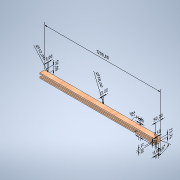
# Autodesk Inventor part: u_lange_Stange
Saved by Autodesk Inventor 2020.3 (Build 243373000, 373)
## iProperties
Created: 2020-09-30
Part Number: u_lange_Stange
Material: Birch
Document SubType Name: Modeling
Designer: Mara
Density: 0.512 g/cm^3
Appearance: Birch - Natural Medium Gloss
Author: Mara
Autodesk Inventor part; units mm, degrees
ref_plane "YZ Plane" through (0, 0, 0) normal (1, 0, 0) x (0, 1, 0)
ref_plane "XZ Plane" through (0, 0, 0) normal (0, 1, 0) x (-1, 0, 0)
ref_plane "XY Plane" through (0, 0, 0) normal (0, 0, 1) x (1, 0, 0)
sketch "Sketch1" plane through (0, 0, 0) normal (0, 0, 1) x (1, 0, 0)
  line L0 (-600, -25) -> (600, -25)
  line L1 (600, -25) -> (600, 25)
  line L2 (600, 25) -> (-600, 25)
  line L3 (-600, 25) -> (-600, -25)
  line L4 (-600, -25) -> (600, 25) construction
  line L5 (600, -25) -> (-600, 25) construction
  point P0 (0, 0)
  dimension "d0" = 1200
  dimension "d1" = 50
  constraints: 12 end point, 2 midpoint, 2 parallel, 1 horizontal, 1 perpendicular
  measures "d0" distance of L2.end L1.end
  measures "d1" distance of L1.end L0.end
extrude "Extrusion1" add sketch "Sketch1" along normal blind 50
sketch "Sketch2" plane through (0, 0, 0) normal (0, 0, -1) x (-1, 0, 0)
  circle A0 centre (0, 0) radius 9
  circle A1 centre (570, 0) radius 6
  line L0 (600, 25) -> (600, -25) projected
  line L1 (-600, 25) -> (600, 25) projected
  dimension "d13" = 18
  dimension "d20" = 30
  dimension "d21" = 12
  dimension "d22" = 50
  dimension "d23" = 25
  constraints: 2 centre point, 1 coincident
  measures "d13" diameter of A0
  measures "d20" distance from line of L0 A1.centre
  measures "d21" diameter of A1
  measures "d22" distance of L0.start L0.end
  measures "d23" distance from line of L1 A1.centre
extrude "Extrusion2" add sketch "Sketch2" along normal blind 13
sketch "Sketch5" plane through (0, 0, 0) normal (0, 0, -1) x (-1, 0, 0)
  line L0 (600, -25) -> (-600, -25) projected
  line L1 (-391, -25) -> (-391, -3)
  line L2 (-391, -3) -> (-380, -3)
  line L3 (-380, -3) -> (-380, -25) construction
  line L4 (-380, -3) -> (-374.1051, -25)
  point P0 (0, 0)
  dimension "d30" = 15
  dimension "d31" = 22
  dimension "d32" = 11
  dimension "d33" = 209
  constraints: 8 end point, 3 point on line, 2 perpendicular, 1 vertical
  measures "d30" angle of L3 L4
  measures "d31" distance between parallel lines of L0 L2
  measures "d32" distance of L1.end L2.end
  measures "d33" distance of L0.end L1.start
extrude "Extrusion4" cut sketch "Sketch5" against normal through all
sketch "Sketch6" plane through (600, -25, 0) normal (1, 0, 0) x (0, 0, -1)
  line L0 (-50, 0) -> (-50, 50) projected
  line L1 (0, 50) -> (-50, 50) projected
  line L2 (0, 0) -> (0, 50) projected
  line L3 (0, 50) -> (-50, 50) projected
  line L4 (-50, 0) -> (-50, 50) projected
  line L5 (0, 0) -> (-50, 0) projected
  line L6 (-50, 36) -> (-39, 36)
  line L7 (-39, 36) -> (-39, 44)
  line L8 (-50, 14) -> (-39, 14)
  line L9 (-39, 14) -> (-39, 6)
  line L10 (-23, 36.8677) -> (-23, 13.1323)
  line L11 (-23, 36.8677) -> (-31.5, 44)
  line L12 (-31.5, 44) -> (-39, 44)
  line L13 (-23, 13.1323) -> (-31.5, 6)
  line L14 (-31.5, 6) -> (-39, 6)
  point P0 (0, 25)
  dimension "d36" = 14
  dimension "d37" = 14
  dimension "d38" = 8
  dimension "d42" = 16
  dimension "d43" = 11
  dimension "d44" = 7.5
  dimension "d88" = 140
  dimension "d89" = 140
  constraints: 18 end point, 4 horizontal, 3 equal length, 2 perpendicular, 2 point on line, 1 vertical
  measures "d36" distance between parallel lines of L1 L6
  measures "d37" distance between parallel lines of L5 L8
  measures "d38" distance of L6.end L7.end
  measures "d42" distance from line of L10 L6.end
  measures "d43" distance of L6.start L6.end
  measures "d44" distance of L11.end L7.end
  measures "d88" angle of L12 L11
  measures "d89" angle of L14 L13
extrude "Extrusion5" cut sketch "Sketch6" against normal through all contours L0 L6 L7 L12 L11 L10 L13 L14 L9 L8
equation "\"d23\" = 0.5 * d22"
equation "\"d37\" = d36"
equation "\"d89\" = d88"
body "Solid1"
